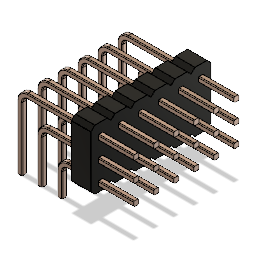
electrical unit 2 (Autodesk Fusion 360 design; units mm, degrees)
Autodesk Fusion 360 part; units mm, degrees
sketch "Sketch1" plane through (0, 0, 0) normal (0, 1, 0) x (1, 0, 0)
  line L0 (0.225, 0.325) -> (-0.225, 0.325)
  line L1 (-0.325, 0.225) -> (-0.325, -0.225)
  line L2 (-0.225, -0.325) -> (0.225, -0.325)
  line L3 (0.325, -0.225) -> (0.325, 0.225)
  line L4 (0.275, 0.275) -> (-0.275, -0.275) construction
  line L5 (-0.275, 0.275) -> (0.275, -0.275) construction
  line L6 (-0.325, 0.225) -> (-0.225, 0.325)
  line L7 (-0.225, -0.325) -> (-0.325, -0.225)
  line L8 (0.325, -0.225) -> (0.225, -0.325)
  line L9 (0.225, 0.325) -> (0.325, 0.225)
  line L10 (2.765, 0.325) -> (2.315, 0.325)
  line L11 (2.215, 0.225) -> (2.215, -0.225)
  line L12 (2.315, -0.325) -> (2.215, -0.225)
  line L13 (2.315, -0.325) -> (2.765, -0.325)
  line L14 (2.865, -0.225) -> (2.865, 0.225)
  line L15 (2.765, 0.325) -> (2.865, 0.225)
  line L16 (2.865, -0.225) -> (2.765, -0.325)
  line L17 (2.215, 0.225) -> (2.315, 0.325)
  line L18 (5.305, 0.325) -> (4.855, 0.325)
  line L19 (4.755, 0.225) -> (4.755, -0.225)
  line L20 (4.855, -0.325) -> (4.755, -0.225)
  line L21 (4.855, -0.325) -> (5.305, -0.325)
  line L22 (5.405, -0.225) -> (5.405, 0.225)
  line L23 (5.305, 0.325) -> (5.405, 0.225)
  line L24 (5.405, -0.225) -> (5.305, -0.325)
  line L25 (4.755, 0.225) -> (4.855, 0.325)
  dimension "d5" = 360
  dimension "d6" = 0.45
  dimension "d9" = 2.54
  dimension "d10" = 0
  constraint horizontal L0
  constraint perpendicular L0 L1
  constraint parallel L0 L2
  constraint parallel L1 L3
  constraint coincident L4 origin
  constraint coincident L5 origin
  constraint coincident L9 L4.start
  constraint coincident L8 L5.end
  constraint coincident L7 L4.end
  constraint coincident L6 L5.start
  measures "d6" distance of L0.end L0.start
sketch "Sketch2" plane through (0, 0, 0) normal (0, 0, 1) x (1, 0, 0)
  line L0 (0, 0) -> (0, 8.08)
  line L1 (1, 9.08) -> (14.48, 9.08)
  line L2 (2.54, 0) -> (2.54, 5.54)
  line L3 (3.54, 6.54) -> (14.48, 6.54)
  line L4 (5.08, 0) -> (5.08, 3)
  line L5 (6.08, 4) -> (14.48, 4)
  arc A0 (1, 9.08) -> (0, 8.08) centre (1, 8.08) ccw
  arc A1 (3.54, 6.54) -> (2.54, 5.54) centre (3.54, 5.54) ccw
  arc A2 (6.08, 4) -> (5.08, 3) centre (6.08, 3) ccw
  point P0 (0, 9.08)
  point P1 (2.54, 6.54)
  dimension "d11" = 9.08
  dimension "d12" = 14.48
  dimension "d13" = 6.54
  dimension "d15" = 1
  constraint coincident L0.start origin
  constraint vertical L0
  constraint perpendicular L0 L1
  constraint perpendicular L2 L3
  constraint perpendicular L4 L5
  constraint vertical L1.end L3.end
  constraint vertical L3.end L5.end
  constraint coincident P0 L0
  constraint coincident P0 L1
  constraint tangent L0 A0
  constraint tangent L1 A0
  constraint coincident P1 L3
  constraint coincident P1 L2
  constraint tangent L3 A1
  constraint tangent L2 A1
  constraint equal A0 A1
  constraint tangent L5 A2
  constraint tangent L4 A2
  constraint equal A0 A2
  measures "d11" distance of L0.start P0
  measures "d12" distance of P0 L1.end
  measures "d13" distance of L2.start P1
  measures "d15" radius of A0
sweep "Sweep1" add profiles "Sketch1" path "Sketch2" along L4 A2 L5 section 1 contours L18 L19 L20 L21 L22 L23 L24 L25 makes body 1
sweep "Sweep2" add profiles "Sketch1" path "Sketch2" along L2 A1 L3 section 1 contours L10 L11 L12 L13 L14 L15 L16 L17 separate body makes body 2
sweep "Sweep3" add profiles "Sketch1" path "Sketch2" along L0 A0 L1 section 1 contours L0 L1 L2 L3 L6 L7 L8 L9 separate body makes body 3
ref_plane "WorkPlane1" through (7.5, 0, 0) normal (1, 0, 0) x (0, 1, 0)
sketch "Sketch3" plane through (7.5, 0, 0) normal (1, 0, 0) x (0, 0, -1)
  line L0 (0, 0) -> (0, 9.405) construction
  line L1 (0.225, 9.405) -> (-0.225, 9.405) construction
  line L2 (0.77, 10.675) -> (-0.77, 10.675)
  line L3 (-1.27, 10.175) -> (-1.27, 3.555)
  line L4 (-0.77, 3.055) -> (0.77, 3.055)
  line L5 (1.27, 3.555) -> (1.27, 10.175)
  line L6 (1.145, 10.3) -> (-1.145, 3.43) construction
  line L7 (-1.27, 10.675) -> (1.27, 3.055) construction
  line L8 (0, 9.405) -> (0.3211, 9.405) construction
  line L9 (0.225, 6.865) -> (-0.225, 6.865) construction
  line L10 (-1.27, 10.175) -> (-0.77, 10.675)
  line L11 (0, 6.865) -> (0, 10.675) construction
  line L12 (-1.27, 6.865) -> (1.27, 6.865) construction
  line L13 (1.27, 10.175) -> (0.77, 10.675)
  line L14 (-1.27, 3.555) -> (-0.77, 3.055)
  line L15 (1.27, 3.555) -> (0.77, 3.055)
  point P0 (0, 6.865)
  dimension "d37" = 1.27
  dimension "d39" = 0.5
  dimension "d40" = 0.5
  constraint coincident L0.start origin
  constraint vertical L0
  constraint midpoint L0.end L1
  constraint horizontal L2
  constraint perpendicular L2 L3
  constraint parallel L2 L4
  constraint parallel L3 L5
  constraint coincident L6 P0
  constraint coincident L7 P0
  constraint coincident L0 P0
  constraint coincident L0 L8.start
  constraint perpendicular L0 L8
  constraint coincident P0 L9
  constraint coincident P0 L11.start
  constraint symmetric L3.start L11 L5.end
  constraint symmetric L2.end L11 L2.start
  constraint symmetric L3.start L12 L3.end
  constraint symmetric L2.end L12 L4.start
  constraint symmetric L12 L5.end L5.start
  constraint symmetric L12 L2.start L4.end
  constraint coincident L3 L12.start
  constraint coincident L2 L11.end
  constraint coincident L13 L6.start
  constraint coincident L5 L12.end
  constraint coincident L14 L6.end
  measures "d37" vertical distance of L7.start L8.end
  measures "d39" distance of L7.start L3.start
  measures "d40" distance of L7.start L2.end
extrude "Extrude1" add sketch "Sketch3" along normal blind 2.5 bodies 1 2 3
pattern_linear "R-Pattern1" count 6 spacing 2.54 along (0, 0, -1) of bodies 1 makes body 4 at (7.5, 6.8317, -1.585) makes body 5 at (7.5, 6.8317, -4.125) makes body 6 at (7.5, 6.8317, -6.665) makes body 7 at (7.5, 6.8317, -9.205) makes body 8 at (7.5, 6.8317, -11.745)
combine "Combine1" operation add target body 1 tool bodies 4 5 8 7 6
